Autodesk Fusion 360 part; units mm, degrees
(part 3 of 3)
  measures "d602" diameter of A109
  measures "d603" diameter of A112
  measures "d604" diameter of A105
  measures "d605" distance of L261.end L261.start
  measures "d606" distance of L264.start L264.end
  measures "d607" distance of P13 P18
  measures "d608" distance of P20 P18
  measures "d609" radius of A93
  measures "d610" radius of A107
  measures "d611" radius of A99
  measures "d612" radius of A101
  measures "d613" radius of A97
  measures "d614" radius of A100
  measures "d615" radius of A103
  measures "d616" radius of A108
  measures "d617" diameter of A94
  measures "d618" diameter of A96
  measures "d807" distance of L290.end L291.start
  measures "d858" radius of A115
  measures "d859" radius of A127
  measures "d860" radius of A114
  measures "d861" radius of A126
  measures "d862" diameter of A117
  measures "d863" diameter of A128
  measures "d865" diameter of A116
  measures "d876" radius of A125
  measures "d877" radius of A118
  measures "d878" radius of A124
  measures "d879" radius of A119
  measures "d880" diameter of A123
  measures "d881" diameter of A121
  measures "d882" diameter of A120
  measures "d883" diameter of A122
  measures "d884" diameter of A129
  measures "d892" radius of A137
  measures "d893" radius of A130
  measures "d894" radius of A136
  measures "d895" radius of A134
  measures "d896" diameter of A132
  measures "d897" diameter of A133
  measures "d898" diameter of A135
  measures "d899" radius of A141
  measures "d900" radius of A145
  measures "d901" radius of A138
  measures "d902" radius of A144
  measures "d903" diameter of A143
  measures "d904" diameter of A139
  measures "d905" diameter of A142
  measures "d906" diameter of A140
  measures "d907" diameter of A131
  measures "d934" distance of L299.end L299.start
  measures "d943" diameter of A146
  measures "d944" diameter of A147
  measures "d945" distance of L288.end L332.end
  measures "d946" distance of L288.end L334.end
  measures "d947" distance of L290.end L336.end
  measures "d948" distance of L290.end L338.end
  measures "d949" distance of L291.start L340.end
  measures "d950" distance of L291.start L342.end
  measures "d951" distance of L292.end L344.end
  measures "d953" diameter of A152
  measures "d954" diameter of A153
  measures "d955" diameter of A154
  measures "d956" diameter of A155
  measures "d957" distance of L360.end L356.end
  measures "d959" distance of L353.start L349.end
  measures "d961" distance of L352.end L356.end
  measures "d962" distance of L361.start L360.end
  measures "d963" distance of L351.end L360.end
  measures "d964" distance of L358.end L349.start
  measures "d965" distance of L350.start L349.start
  measures "d966" diameter of A156
  measures "d967" diameter of A157
  measures "d968" diameter of A158
  measures "d969" diameter of A159
  measures "d981" distance of L102.start L372.end
  measures "d983" distance of L102.end L376.end
  measures "d1011" diameter of A160
  measures "d1012" diameter of A166
  measures "d1013" diameter of A163
  measures "d1014" diameter of A161
  measures "d1015" diameter of A165
  measures "d1016" diameter of A164
  measures "d1017" diameter of A162
  measures "d1018" distance of L379.start L381.start
  measures "d1019" distance of L381.start L380.start
  measures "d1020" distance of L381.start L382.start
  measures "d1037" diameter of A172
  measures "d1038" diameter of A170
  measures "d1039" diameter of A169
  measures "d1040" diameter of A167
  measures "d1041" diameter of A173
  measures "d1042" diameter of A171
  measures "d1043" diameter of A168
  measures "d1044" distance of L387.end L389.start
  measures "d1045" distance of L387.end L386.start
  measures "d1046" distance of L387.end L388.start
  measures "d1047" distance of L389.end L390.end
  measures "d1048" distance of L389.end L393.start
  measures "d1049" distance of L379.start L378.start
  measures "d1050" distance of L378.end L378.start
  measures "d1051" distance of L378.start L398.end
  measures "d1052" distance of L378.start L400.end
  measures "d1055" radius of A174
  measures "d1056" radius of A177
  measures "d1057" distance of L406.start L399.end
  measures "d1058" distance of L406.start L380.end
  measures "d1059" diameter of A184
  measures "d1060" diameter of A181
  measures "d1061" diameter of A188
  measures "d1062" diameter of A187
  measures "d1063" diameter of A182
  measures "d1064" diameter of A185
  measures "d1065" diameter of A186
  measures "d1066" distance of L411.start L411.end
  measures "d1069" distance of L416.end L411.end
  measures "d1072" radius of A178
  measures "d1073" radius of A183
  measures "d1074" distance of L416.end L418.end
  measures "d1075" distance of L416.end L420.end
  measures "d1076" distance of L411.start L422.end
  measures "d1077" distance of L411.start L424.end
  measures "d1094" diameter of A203
  measures "d1095" diameter of A205
  measures "d1096" diameter of A198
  measures "d1097" diameter of A200
  measures "d1098" diameter of A190
  measures "d1099" diameter of A194
  measures "d1100" diameter of A193
  measures "d1101" diameter of A196
  measures "d1102" diameter of A189
  measures "d1103" distance of L427.start L427.end
  measures "d1104" distance of L430.end L427.end
  measures "d1105" radius of A192
  measures "d1106" radius of A199
  measures "d1107" distance of L433.end L430.end
  measures "d1108" distance of L430.end L426.end
  measures "d1109" distance of L439.end L427.start
  measures "d1110" distance of L429.start L427.start
  measures "d1111" diameter of A213
  measures "d1112" diameter of A216
  measures "d1113" diameter of A208
  measures "d1114" diameter of A210
  measures "d1115" diameter of A211
  measures "d1116" diameter of A215
  measures "d1117" diameter of A214
  measures "d1118" distance of L460.end L451.start
  measures "d1119" distance of L460.end L461.end
  measures "d1120" distance of L460.end L463.start
  measures "d1121" distance of L451.end L451.start
  measures "d1122" distance of L451.end L455.start
  measures "d1123" distance of L448.end L451.end
  measures "d1124" radius of A212
  measures "d1125" radius of A209
  measures "d1126" distance of L462.end L448.start
  measures "d1127" distance of L462.end L459.end
  measures "d1144" distance of L469.end L470.end
  measures "d1145" distance of L468.end L469.end
  measures "d1146" distance of L475.end L476.end
  measures "d1147" distance of L474.end L475.end
  measures "d1148" radius of A220
  measures "d1171" distance of L497.start L487.start
  measures "d1174" distance of L487.start L490.start
  measures "d1187" distance of L485.start L485.end
  measures "d1188" distance of L485.start L481.end
  measures "d1189" distance of L480.start L513.end
  measures "d1190" distance of L497.start L502.end
  measures "d1191" distance of L487.start L487.end
  measures "d1192" distance of L487.start L498.start
  measures "d1193" diameter of A223
  measures "d1194" diameter of A218
  measures "d1195" diameter of A219
  measures "d1196" diameter of A217
  measures "d1197" distance of L485.start L487.start
  measures "d1210" distance of L486.end L489.start
  measures "d1211" distance of L486.end L486.start
  measures "d1212" distance of L483.end L484.end
  measures "d1213" distance of L483.start L484.end
  measures "d1237" distance of L527.end L525.start
  measures "d1253" distance of L517.start L516.start
  measures "d1254" distance of L517.start L518.end
  measures "d1255" distance of L519.end L519.start
  measures "d1256" distance of L527.end L530.end
  measures "d1257" distance of L525.start L533.end
  measures "d1258" distance of L525.start L534.end
  measures "d1259" diameter of A227
  measures "d1260" diameter of A225
  measures "d1261" diameter of A226
  measures "d1262" diameter of A224
  measures "d1263" distance of L517.start L525.start
  measures "d1322" distance of L538.end L539.end
  measures "d1323" distance of L537.end L538.end
  measures "d1324" distance of L544.end L545.end
  measures "d1325" distance of L543.end L544.end
  measures "d1326" distance of L559.end L560.end
  measures "d1327" distance of L558.end L559.end
  measures "d1328" distance of L565.end L566.end
  measures "d1329" distance of L564.end L565.end
  measures "d1330" distance of L571.end L572.end
  measures "d1331" distance of L570.end L571.end
  measures "d1332" distance of L602.start L602.end
  measures "d1333" distance of L615.start L615.end
  measures "d1334" distance of L602.start L615.end
  measures "d1335" distance of P72 L599.end
  measures "d1336" distance of P72 L598.start
  measures "d1337" distance of L601.end L597.end
  measures "d1338" distance of L597.start L597.end
  measures "d1339" distance of L596.end L610.end
  measures "d1340" distance of L596.start L610.end
extrude "돌출62" add sketch "스케치1" along normal blind 5 contours L495 L497 L510 L511 makes body 1
extrude "돌출63" add sketch "스케치1" along normal blind 9 separate body contours L30 L31 L32 L33 | L102 L103 L104 L105 | L106 L107 L108 L109 | L174 L176 L178 L183 | L202 L203 L204 L205 | L206 L207 L208 L209 | L210 L211 L212 L213 | L214 L215 L216 L217 | L218 L219 L220 L221 | L222 L223 L224 L225 | L226 L227 L228 L229 | L230 L231 L232 L233 | L288 L289 L290 L291 L292 L293 | L296 L303 L306 L307 | L310 L311 L313 L321 | L326 L327 L328 L329 L330 | L349 L356 L362 L365 L366 L368 | L406 L407 L408 L409 | L432 L438 L441 L443 L445 | L453 L459 L462 L466 | L524 L526 L527 L528 makes body 2 at (1528.4276, -1089.433, 0) makes body 3 at (813.4968, -867.598, 0) makes body 4 at (1340.4245, -1498.5046, 0) makes body 5 at (624.4965, -1590.7079, 0) makes body 6 at (435.1019, 338.1172, 0) makes body 7 at (241.3333, -481, 0) makes body 8 at (264.4965, -1590.7079, 0) makes body 9 at (1170.9143, -1085.7127, 0) makes body 10 at (1163.4968, -867.598, 0) makes body 11 at (1550.7609, -1439.433, 0) makes body 12 at (1751.5009, -955.9592, 0) makes body 13 at (1428.4276, -1089.433, 0) makes body 14 at (813.4968, -1667.598, 0) makes body 15 at (990.4245, -1498.5046, 0) makes body 16 at (50.5, -1292, 0) makes body 17 at (348.4329, -826.6931, 0) makes body 18 at (221.3333, -1446.3333, 0) makes body 19 at (820.9143, -1085.7127, 0) makes body 20 at (1163.4968, -1667.598, 0) makes body 21 at (1450.7609, -1439.433, 0) makes body 22 at (1811.5009, -1585.9592, 0)
move_body "정렬110" bodies 7 to x (1, 0, 0) y (0, 1, 0) z (0, 0, 1) at (0, 725, 9)
move_body "이동82" bodies 16 8 5 18 to x (1, 0, 0) y (0, 0, 1) z (0, -1, 0) at (0, -1213.5, 1218.5)
move_body "이동83" bodies 5 8 to x (0, -1, 0) y (1, 0, 0) z (0, 0, 1) at (1446.3298, -980.6702, 0)
move_body "정렬111" bodies 5 to x (1, 0, 0) y (0, 1, 0) z (0, 0, 1) at (431.1702, 1862, 426.7079)
move_body "정렬112" bodies 8 to x (1, 0, 0) y (0, 1, 0) z (0, 0, 1) at (-223.8298, 1502, 426.7079)
move_body "정렬113" bodies 16 to x (1, 0, 0) y (0, 1, 0) z (0, 0, 1) at (0, 1738.5, 132.5)
move_body "정렬114" bodies 18 to x (1, 0, 0) y (0, 1, 0) z (0, 0, 1) at (0, 1456.5, 294.5)
move_body "정렬115" bodies 17 to x (1, 0, 0) y (0, 1, 0) z (0, 0, 1) at (0, 1100, 91)
move_body "정렬116" bodies 1 to x (1, 0, 0) y (0, 1, 0) z (0, 0, 1) at (0, 1450, 100)
move_body "이동84" bodies 3 10 12 20 22 9 4 19 15 14 to x (0, -1, 0) y (1, 0, 0) z (0, 0, 1) at (1628.7615, -195.7679, 0)
move_body "이동85" bodies 12 15 19 4 9 22 to x (0, 0, 1) y (0, 1, 0) z (-1, 0, 0) at (630.3286, 0, -630.3286)
move_body "정렬117" bodies 22 to x (1, 0, 0) y (0, 1, 0) z (0, 0, 1) at (-9, 569.5041, 317.5262)
move_body "정렬118" bodies 10 to x (1, 0, 0) y (0, 1, 0) z (0, 0, 1) at (-171.1683, 0, -280)
move_body "정렬119" bodies 4 to x (1, 0, 0) y (0, 1, 0) z (0, 0, 1) at (-85, 0, 339)
move_body "정렬120" bodies 15 to x (1, 0, 0) y (0, 1, 0) z (0, 0, 1) at (42.6714, 1437.2647, 619)
move_body "정렬121" bodies 14 to x (1, 0, 0) y (0, 1, 0) z (0, 0, 1) at (756.5032, 1437.2647, 0)
move_body "정렬122" bodies 12 to x (1, 0, 0) y (0, 1, 0) z (0, 0, 1) at (118.6714, 2356.7688, 247.5262)
move_body "정렬123" bodies 19 to x (1, 0, 0) y (0, 1, 0) z (0, 0, 1) at (127.6714, 1437.2647, 280)
move_body "정렬124" bodies 20 to x (1, 0, 0) y (0, 1, 0) z (0, 0, 1) at (756.5032, 1787.2647, 291)
move_body "정렬125" bodies 4 to x (1, 0, 0) y (0, 1, 0) z (0, 0, 1) at (-545.3286, 1787.2647, 280)
move_body "정렬126" bodies 10 to x (1, 0, 0) y (0, 1, 0) z (0, 0, 1) at (-621.3286, 1787.2647, 280)
move_body "정렬127" bodies 22 to x (1, 0, 0) y (0, 1, 0) z (0, 0, 1) at (-697.3286, 1787.2647, 280)
move_body "정렬128" bodies 9 to x (1, 0, 0) y (0, 1, 0) z (0, 0, 1) at (-715.3286, 1787.2647, 280)
move_body "정렬129" bodies 3 to x (1, 0, 0) y (0, 1, 0) z (0, 0, 1) at (-792.4968, 1437.2647, 291)
move_body "이동86" bodies 11 13 21 2 to x (1, 0, 0) y (0, 0, 1) z (0, -1, 0) at (0, -1481.933, 1490.933)
move_body "정렬130" bodies 21 to x (1, 0, 0) y (0, 1, 0) z (0, 0, 1) at (-733.0943, 1724.933, 145.5)
move_body "정렬131" bodies 11 to x (1, 0, 0) y (0, 1, 0) z (0, 0, 1) at (-833.0943, 2006.933, 145.5)
move_body "정렬132" bodies 2 to x (1, 0, 0) y (0, 1, 0) z (0, 0, 1) at (-1582.0943, 2006.933, -204.5)
move_body "정렬133" bodies 13 to x (1, 0, 0) y (0, 1, 0) z (0, 0, 1) at (-1482.0943, 1724.933, -204.5)
equation "d1077 = 26.5 mm - 9 mm"
